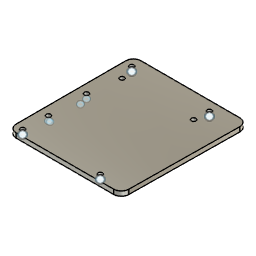
1st layer rear (Autodesk Fusion 360 design; units mm, degrees)
Autodesk Fusion 360 part; units mm, degrees
sketch "Sketch1" plane through (0, 0, 0) normal (0, 0, 1) x (1, 0, 0)
sketch "Sketch1 (2)" plane through (0, 0, 0) normal (0, 0, 1) x (1, 0, 0) in component "Car Fram v4 v1"
  line L0 (15, 5) -> (15, 77)
  line L1 (20, 82) -> (69, 82)
  line L2 (20, 0) -> (69, 0)
  circle A0 centre (20.1, 75.85) radius 1.5
  circle A1 centre (71.1, 75.85) radius 1.5
  circle A2 centre (20.1, 4.15) radius 1.5
  circle A3 centre (71.1, 4.15) radius 1.5
  arc A4 (20, 82) -> (15, 77) centre (20, 77) ccw
  arc A5 (15, 5) -> (20, 0) centre (20, 5) ccw
  line L3 (69, 82) -> (70, 82)
  line L4 (70, 0) -> (69, 0)
  circle A6 centre (23.7662, 65.8232) radius 1.5
  circle A7 centre (70.7662, 65.8232) radius 1.5
  line L5 (69, 0) -> (84.0606, 0)
  line L6 (70, 82) -> (84.9387, 82)
  line L7 (89.0602, 4.939) -> (89.9383, 76.939)
  arc A8 (84.0606, 0) -> (89.0602, 4.939) centre (84.0606, 5) ccw
  arc A9 (89.9383, 76.939) -> (84.9387, 82) centre (84.9387, 77) ccw
  point P0 (15, 0)
  point P1 (15, 82)
  point P2 (89, 0)
  point P3 (90, 82)
  dimension "d20_5" = 54
  dimension "d21_4" = 54
  dimension "d22_4" = 3
  dimension "d23_3" = 3
  dimension "d24_3" = 6.15
  dimension "d25_3" = 6.15
  dimension "d26_3" = 5.1
  dimension "d27_3" = 51
  dimension "d56_5" = 82
  dimension "d68_4" = 5
  dimension "d69_4" = 5
  dimension "d76_4" = 71.7
  dimension "d77_4" = 71.7
  dimension "d5_3" = 3
  dimension "d6_4" = 3
  dimension "d428" = 20
  dimension "d430" = 20
  dimension "d431" = 5
  constraint perpendicular L0 L1
  constraint perpendicular L0 L2
  constraint coincident P1 L0
  constraint coincident P1 L1
  constraint tangent L0 A4
  constraint tangent L1 A4
  constraint coincident P0 L0
  constraint coincident P0 L2
  constraint tangent L0 A5
  constraint tangent L2 A5
  constraint horizontal L3
  constraint parallel L3 L4
  constraint parallel L4 L5
  constraint horizontal L6
  constraint coincident P2 L5
  constraint coincident P2 L7
  constraint tangent L5 A8
  constraint tangent L7 A8
  constraint coincident P3 L7
  constraint coincident P3 L6
  constraint tangent L7 A9
  constraint tangent L6 A9
  constraint equal A8 A9
  measures "d20_5" distance of P1 L1.end
  measures "d21_4" distance of P0 L2.end
  measures "d22_4" diameter of A0
  measures "d23_3" diameter of A1
  measures "d24_3" distance of L1 A0.centre
  measures "d25_3" distance of L1 A1.centre
  measures "d26_3" distance of L0 A0.centre
  measures "d27_3" distance of A0.centre A1.centre
  measures "d56_5" distance of P0 P1
  measures "d68_4" radius of A4
  measures "d69_4" radius of A5
  measures "d76_4" distance of A0.centre A2.centre
  measures "d77_4" distance of A1.centre A3.centre
  measures "d5_3" diameter of A6
  measures "d6_4" diameter of A7
  measures "d428" distance of L2.end P2
  measures "d430" distance of L3.end P3
  measures "d431" radius of A8
extrude "Extrude3" add sketch "Sketch1 (2)" along normal blind 3 makes body 1 in component "Car Fram v4 v1"
extrude "Extrude4" add sketch "Sketch1 (2)" along normal blind 3 separate body makes body 2 in component "Car Fram v4 v1"
sketch "sketch 1333" plane through (109.8228, 84.0241, 0) normal (0, 0, -1) x (1, 0, 0)
  circle A0 centre (-89.7228, 79.8741) radius 1.5
  circle A1 centre (-89.7228, 79.8741) radius 1.5
  circle A2 centre (-89.7228, 79.8741) radius 2
  circle A3 centre (-38.7228, 8.1741) radius 1.5
  circle A4 centre (-38.7228, 8.1741) radius 1.5
  circle A5 centre (-38.7228, 8.1741) radius 2
  circle A6 centre (-38.7228, 79.8741) radius 1.5
  circle A7 centre (-38.7228, 79.8741) radius 1.5
  circle A8 centre (-38.7228, 79.8741) radius 2
  circle A9 centre (-89.7228, 8.1741) radius 1.5
  circle A10 centre (-89.7228, 8.1741) radius 1.5
  circle A11 centre (-89.7228, 8.1741) radius 2
extrude "Extrude5" add sketch "sketch 1333" along normal blind 50 bodies 1 2 in component "Car Fram v4 v1"
delete_face "DeleteFace1" 1 faces at (22.0901, 76.0491, -16.6667) on bodies 1 in component "Car Fram v4 v1"
delete_face "DeleteFace2" 1 faces at (72.8564, 74.8935, -33.3333) on bodies 1 in component "Car Fram v4 v1"
delete_face "DeleteFace3" 1 faces at (72.6321, 2.8644, -33.3333) on bodies 1 in component "Car Fram v4 v1"
delete_face "DeleteFace4" 1 faces at (22.0901, 4.3491, -16.6667) on bodies 1 in component "Car Fram v4 v1"
sketch "sketch 1388" plane through (109.8228, -24.5923, 0) normal (0, 0, -1) x (0, 1, 0)
  circle A0 centre (28.7423, -38.7228) radius 1.5
  circle A1 centre (28.7423, -38.7228) radius 2
  circle A2 centre (100.4423, -38.7228) radius 1.5
  circle A3 centre (100.4423, -38.7228) radius 2
  circle A4 centre (100.4423, -89.7228) radius 1.5
  circle A5 centre (100.4423, -89.7228) radius 2
  circle A6 centre (28.7423, -89.7228) radius 1.5
  circle A7 centre (28.7423, -89.7228) radius 2
extrude "Extrude6" add sketch "sketch 1388" along normal blind 34 bodies 1 in component "Car Fram v4 v1"
sketch "sketch 1430" plane through (109.8228, -24.5923, 0) normal (0, 0, -1) x (0, 1, 0)
  circle A0 centre (45, -88) radius 1.5
  circle A1 centre (65, -88) radius 1.5
extrude "Extrude7" cut sketch "sketch 1430" against normal blind 5 bodies 1 in component "Car Fram v4 v1"
delete_face "DeleteFace5" 1 faces at (21.6734, 41.9002, 1) on bodies 1 in component "Car Fram v4 v1"
delete_face "DeleteFace6" 1 faces at (21.8975, 21.9058, 1) on bodies 1 in component "Car Fram v4 v1"
sketch "sketch 1452" plane through (109.8228, -24.5923, 0) normal (0, 0, -1) x (0, 1, 0)
  circle A0 centre (45, -89) radius 1.5
  circle A1 centre (70, -89) radius 1.5
extrude "Extrude8" cut sketch "sketch 1452" against normal blind 5 bodies 1 in component "Car Fram v4 v1"
delete_face "DeleteFace7" 1 faces at (71.1997, 2.1525, -22.6667) on bodies 1 in component "Car Fram v4 v1"
delete_face "DeleteFace8" 1 faces at (71.4963, 77.8103, -22.6667) on bodies 1 in component "Car Fram v4 v1"
delete_face "DeleteFace9" 1 faces at (20.0003, 77.8475, -22.6667) on bodies 1 in component "Car Fram v4 v1"
delete_face "DeleteFace10" 1 faces at (20.1997, 6.1475, -11.3333) on bodies 1 in component "Car Fram v4 v1"
component "Car Fram v4 v1" placed x (1, 0, 0) y (0, 1, 0) z (0, 0, 1) at (0, 0, 0)
